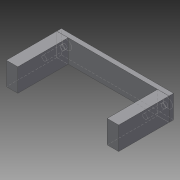
# Autodesk Inventor part: ArOZ Portable support
Saved by Autodesk Inventor 2015 (Build 190159000, 159)
## iProperties
Created: 2019-05-11
Part Number: ArOZ Portable support
Material: Generic
Document SubType Name: Modeling
Designer: Toby
Density: 1 g/cm^3
Appearance: Default
Author: Toby
Autodesk Inventor part; units mm, degrees
ref_plane "YZ Plane" through (0, 0, 0) normal (1, 0, 0) x (0, 1, 0)
ref_plane "XZ Plane" through (0, 0, 0) normal (0, 1, 0) x (-1, 0, 0)
ref_plane "XY Plane" through (0, 0, 0) normal (0, 0, 1) x (1, 0, 0)
sketch "Sketch1" plane through (0, 0, 0) normal (0, 0, 1) x (1, 0, 0)
  line L0 (-18.0104, 8.2073) -> (20.9896, 8.2073)
  line L1 (20.9896, 8.2073) -> (20.9896, -13.7927)
  line L2 (20.9896, -13.7927) -> (-18.0104, -13.7927)
  line L3 (-18.0104, -13.7927) -> (-18.0104, 8.2073)
  line L4 (-23.0104, -13.7927) -> (25.9896, -13.7927)
  line L5 (25.9896, -13.7927) -> (25.9896, 10.2073)
  line L6 (25.9896, 10.2073) -> (-23.0104, 10.2073)
  line L7 (-23.0104, 10.2073) -> (-23.0104, -13.7927)
  point P0 (0, 0)
  dimension "d0" = 22
  dimension "d1" = 39
  dimension "d2" = 5
  dimension "d3" = 5
  dimension "d4" = 2
  constraints: 16 end point, 4 parallel, 2 horizontal, 2 perpendicular, 1 collinear
  measures "d0" distance between parallel lines of L2 L0
  measures "d1" distance between parallel lines of L1 L3
  measures "d2" distance between parallel lines of L1 L5
  measures "d3" distance between parallel lines of L3 L7
  measures "d4" distance between parallel lines of L0 L6
extrude "Extrusion1" add sketch "Sketch1" along normal blind 10 contours L3 L4 L7 L6 L5 L1 L0
sketch "Sketch2" plane through (-23.0104, 10.2073, 0) normal (0, 1, 0) x (1, 0, 0)
  line L0 (0, 0) -> (0, -10) projected
  line L1 (49, 0) -> (49, -10) projected
  point P0 (23.0104, 0)
  point P1 (2.5, -5)
  point P2 (46.5, -5)
  dimension "d7" = 2.5
  dimension "d8" = 2.5
  measures "d7" distance from line of L0 point (2.5, -5)
  measures "d8" distance from line of L1 point (46.5, -5)
hole "Hole1" at (-20.5104, 10.2073, 5) at (23.4896, 10.2073, 5) direction (0, -1, 0) diameter 2 depth 10 tip angle 118 countersink diameter 4 countersink angle 90
sketch "Sketch3" plane through (0, 0, 10) normal (0, 0, 1) x (1, 0, 0)
  line L0 (-23.0104, 10.2073) -> (-23.0104, -13.7927) projected
  line L1 (-23.0104, 8.2073) -> (25.9896, 8.2073)
  line L2 (25.9896, 8.2073) -> (25.9896, 8.1973)
  line L3 (25.9896, 8.1973) -> (-23.0104, 8.1973)
  line L4 (-23.0104, 8.1973) -> (-23.0104, 8.2073)
  line L5 (25.9896, -13.7927) -> (25.9896, 10.2073) projected
  line L6 (-18.0104, 8.2073) -> (20.9896, 8.2073) projected
  point P0 (0, 0)
  dimension "d16" = 0.01
  constraints: 8 end point, 2 collinear, 2 parallel, 1 horizontal, 1 perpendicular, 1 point on line
  measures "d16" distance between parallel lines of L1 L3
extrude "Extrusion2" cut sketch "Sketch3" against normal blind 10
body "Solid1"
